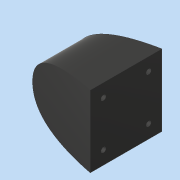
# Autodesk Inventor part: Fore
Saved by Autodesk Inventor 2018 (Build 220112000, 112)
## iProperties
Created: 2017-02-01
Part Number: Fore
Material: ABS Plastic
Document SubType Name: Modeling
Designer: techn
Density: 1.06 g/cm^3
Appearance: Smooth - Black
Author: techn
Autodesk Inventor part; units mm, degrees
ref_plane "YZ Plane" through (0, 0, 0) normal (1, 0, 0) x (0, 1, 0)
ref_plane "XZ Plane" through (0, 0, 0) normal (0, 1, 0) x (-1, 0, 0)
ref_plane "XY Plane" through (0, 0, 0) normal (0, 0, 1) x (1, 0, 0)
sketch "Sketch1" plane through (0, 0, 0) normal (0, 0, 1) x (1, 0, 0)
  line L0 (0, 0) -> (0, 37.846)
  line L1 (0, 18.923) -> (-38.1, 18.923)
  line L2 (0, 37.846) -> (-38.1, 37.846) construction
  line L3 (-38.1, 37.846) -> (-38.1, 18.923) construction
  spline S0 degree 2 poles (0, 37.846) (-38.1, 37.846) (-38.1, 18.923) knots 1 1 1 2 2 2
  line L4 (0, 0) -> (-38.1, 0) construction
  line L5 (-38.1, 0) -> (-38.1, 18.923) construction
  spline S1 degree 2 poles (0, 0) (-38.1, 0) (-38.1, 18.923) knots 1 1 1 2 2 2
  dimension "d0" = 37.846
  dimension "d1" = 38.1
  constraints: 4 end point, 2 perpendicular, 1 horizontal, 1 midpoint, 1 symmetric about line, 1 vertical, 6 other
  measures "d0" distance of L0.start L0.end
  measures "d1" distance of L1.start L1.end
extrude "Extrusion1" add sketch "Sketch1" along normal blind 37.846
sketch "Sketch2" plane through (0, 0, 0) normal (0, 1, 0) x (-1, 0, 0)
  line L0 (38.1, 0) -> (38.1, 37.846) projected
  line L1 (38.1, 0) -> (38.1, 7.62)
  line L2 (0, 0) -> (0, 37.846) projected
  line L3 (38.1, 7.62) -> (0, 0)
  line L4 (0, 0) -> (38.1, 0)
  line L5 (38.1, 37.846) -> (38.1, 30.226)
  line L6 (38.1, 30.226) -> (0, 37.846)
  line L7 (0, 37.846) -> (38.1, 37.846)
  dimension "d4" = 7.62
  dimension "d5" = 7.62
  constraints: 12 end point, 2 perpendicular, 1 point on line
  measures "d4" distance of L0.start L1.end
  measures "d5" distance of L0.end L5.end
extrude "Extrusion11" cut sketch "Sketch2" along normal through all contours L4 L3 L0 | L6 L7 L0
shell "Shell2" thickness 2.54 removed faces 0
sketch "Sketch7" plane through (0, 0, 0) normal (1, 0, 0) x (0, 0, -1)
  line L0 (0, 0) -> (0, 37.846) projected
  line L1 (0, 37.846) -> (-37.846, 37.846) projected
  line L2 (-37.846, 0) -> (-37.846, 37.846) projected
  line L3 (0, 0) -> (-37.846, 0) projected
  line L4 (-34.544, 34.544) -> (-3.302, 34.544)
  line L5 (-3.302, 34.544) -> (-3.302, 3.302)
  line L6 (-3.302, 3.302) -> (-34.544, 3.302)
  line L7 (-34.544, 3.302) -> (-34.544, 34.544)
  circle A0 centre (-30.861, 6.985) radius 1.27
  circle A1 centre (-30.861, 30.861) radius 1.27
  circle A2 centre (-6.985, 6.985) radius 1.27
  circle A3 centre (-6.985, 30.861) radius 1.27
  dimension "d58" = 3.302
  dimension "d59" = 2.54
  dimension "d60" = 6.985
  dimension "d61" = 6.985
  dimension "d64" = 23.876
  dimension "d67" = 23.876
  constraints: 8 end point, 4 centre point, 1 horizontal, 1 vertical, 9 other
  measures "d58" distance between parallel lines of L1 L4
  measures "d59" diameter of A0
  measures "d60" distance from line of L3 A0.centre
  measures "d61" distance from line of A0.centre L2
  measures "d64" distance of A0.centre A1.centre
  measures "d67" distance of A0.centre A2.centre
extrude "Extrusion12" cut sketch "Sketch7" against normal blind 3.175 contours A0 | A1 | A2 | A3
body "Solid1"
